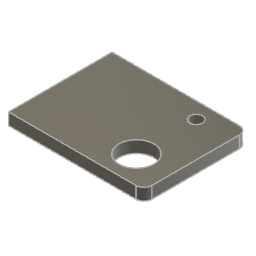
FinalCSProject3 v3 (Autodesk Fusion 360 design; units mm, degrees)
Autodesk Fusion 360 part; units mm, degrees
sketch "Sketch1" plane through (0, 0, 0) normal (0, 1, 0) x (1, 0, 0)
  line L0 (0, 0) -> (85, 0)
  line L1 (85, 0) -> (85, 65)
  line L2 (85, 65) -> (0, 65)
  line L3 (0, 65) -> (0, 0)
  line L4 (0, 17.25) -> (63, 17.25) construction
  line L5 (63, 17.25) -> (63, 0) construction
  line L6 (63, 17.25) -> (63, 65) construction
  line L7 (63, 17.25) -> (63, 54.75)
  circle A0 centre (63, 17.25) radius 11
  circle A1 centre (63, 54.75) radius 4
  line L8 (63, 6.25) -> (63, 0)
  dimension "d1" = 85
  dimension "d2" = 65
  dimension "d4" = 63
  dimension "d5" = 37.5
  dimension "d6" = 22
  dimension "d7" = 8
  dimension "d9" = 6.25
  constraint horizontal L0
  constraint vertical L1
  constraint horizontal L2
  constraint vertical L3
  constraint coincident L0.start L3.end
  constraint coincident L3 L4.start
  constraint perpendicular L3 L4
  constraint coincident L0 L5.end
  constraint perpendicular L0 L5
  constraint coincident L2 L6.end
  constraint perpendicular L2 L6
  constraint perpendicular L4 L7
  constraint coincident L4.end L5.start
  constraint coincident L7.end A1.centre
  constraint coincident A0 L8.start
  constraint coincident L5 L8.start
  measures "d1" distance of L0.start L0.end
  measures "d2" distance of L0.start L2.end
  measures "d4" distance of L4.start L4.end
  measures "d5" distance of L4.end L7.end
  measures "d6" diameter of A0
  measures "d7" diameter of A1
  measures "d9" distance of L5.end L8.start
extrude "Extrude1" add sketch "Sketch1" along normal blind 7.5
fillet "Fillet1" radius 5 1 edges at (85, 3.75, 0)
fillet "Fillet2" radius 5 1 edges at (85, 3.75, -65)
